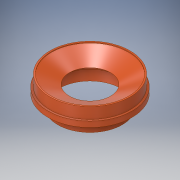
# Autodesk Inventor part: phenolic_top
Saved by Autodesk Inventor 2017 SP1 (Build 210196100, 196)
## iProperties
Created: 2016-07-25
Part Number: phenolic_top
Material: Phenolic Resin
Document SubType Name: Modeling
Designer: Jared
Density: 1.38 g/cm^3
Appearance: Smooth - Light Orange
Author: Jared
Autodesk Inventor part; units mm, degrees
ref_plane "YZ Plane" through (0, 0, 0) normal (1, 0, 0) x (0, 1, 0)
ref_plane "XZ Plane" through (0, 0, 0) normal (0, 1, 0) x (-1, 0, 0)
ref_plane "XY Plane" through (0, 0, 0) normal (0, 0, 1) x (1, 0, 0)
sketch "Sketch1" plane through (0, 0, 0) normal (0, 0, 1) x (1, 0, 0)
  line L0 (0, 25.4) -> (-28.702, 25.4) construction
  line L1 (0, 25.4) -> (-95.25, 25.4) construction
  line L2 (-95.25, 25.4) -> (-90.805, 25.4) construction
  line L3 (-90.805, 25.4) -> (-90.805, 22.4389) construction
  line L4 (-90.805, 0) -> (-95.25, 0)
  line L5 (-28.702, 59.6457) -> (-28.702, -91.9304) construction
  arc A0 (-28.9184, -9.248) -> (-32.3684, -1.8494) centre (-35.052, -7.6045) ccw
  line L6 (-76.2, -185.7054) -> (-28.702, -8.4405)
  line L7 (-90.805, 25.4) -> (-90.805, 0)
  line L8 (-87.63, 23.9195) -> (-32.3684, -1.8494)
  line L9 (-28.702, -7.6045) -> (-60.452, -7.6045) construction
  line L10 (-60.452, -126.9331) -> (-54.102, -126.9331) construction
  line L11 (-54.102, -126.9331) -> (-54.102, -103.2346) construction
  line L12 (-54.102, -103.2346) -> (-60.452, -103.2346)
  line L13 (-60.452, 11.2462) -> (-60.452, 1.7212) construction
  line L14 (-60.452, 11.2462) -> (-60.452, 4.7154) construction
  line L15 (-60.452, 4.7154) -> (-46.4468, 4.7154)
  line L16 (-95.25, 0) -> (-95.25, -12.7) construction
  line L17 (-60.452, -12.7) -> (-73.152, -12.7) construction
  line L18 (-95.25, -12.7) -> (-95.25, -25.4) construction
  line L19 (-95.25, -25.4) -> (-95.25, -88.9) construction
  line L20 (-95.25, -88.9) -> (-82.55, -88.9) construction
  line L21 (-82.55, -88.9) -> (-82.55, -25.4) construction
  line L22 (-95.25, -25.4) -> (-82.55, -25.4)
  line L23 (-82.55, -25.4) -> (-82.55, -88.9)
  line L24 (-82.55, -88.9) -> (-95.25, -88.9)
  line L25 (-95.25, -12.7) -> (-73.152, -12.7)
  line L26 (-73.152, -138.7824) -> (-63.627, -138.7824)
  line L27 (-82.55, -88.9) -> (-82.55, -185.7054)
  line L28 (-82.55, -185.7054) -> (-76.2, -185.7054)
  line L29 (-73.152, -12.7) -> (-73.152, -138.7824)
  line L30 (-88.9, -25.4) -> (-88.9, -31.3436)
  line L31 (-88.9, -31.3436) -> (-95.25, -31.3436)
  line L32 (-95.25, 0) -> (-95.25, -25.4)
  line L33 (-95.25, -31.3436) -> (-95.25, -88.9)
  line L34 (-88.9, -160.3054) -> (-88.9, -221.2532)
  line L35 (-28.9184, -9.248) -> (-85.725, -221.2532)
  line L36 (-85.725, -221.2532) -> (-88.9, -221.2532)
  line L37 (-82.55, -160.3054) -> (-88.9, -160.3054)
  line L38 (-66.802, -38.1) -> (-66.802, 4.7154)
  line L39 (-66.802, 4.7154) -> (-60.452, 4.7154)
  line L40 (-66.802, -38.1) -> (-60.452, -103.2346)
  line L41 (-60.452, 11.2462) -> (-60.452, 4.7154) construction
  line L42 (-60.452, -7.6045) -> (-60.452, -12.7) construction
  line L43 (-60.452, -103.2346) -> (-60.452, -126.9331) construction
  line L44 (0, 59.6457) -> (0, -91.9304) construction
  line L45 (-73.152, -38.1) -> (-69.977, -38.1)
  line L46 (-69.977, -38.1) -> (-69.977, -12.7)
  line L47 (-66.802, -12.7) -> (-69.977, -12.7)
  line L48 (-90.805, 25.4) -> (-87.63, 25.4)
  line L49 (-87.63, 25.4) -> (-87.63, 23.9195)
  point P0 (0, 0)
  point P1 (-95.25, -255.9127)
  point P2 (-88.7095, 22.4389)
  dimension "d0" = 28.702
  dimension "d1" = 95.25
  dimension "d2" = 4.445
  dimension "d5" = 25.4
  dimension "d6" = 25.4
  dimension "d8" = 12.7
  dimension "d12" = 31.75
  dimension "d13" = 6.35
  dimension "d16" = 12.7
  dimension "d17" = 12.7
  dimension "d18" = 12.7
  dimension "d19" = 63.5
  dimension "d20" = 12.7
  dimension "d22" = 9.525
  dimension "d23" = 6.35
  dimension "d25" = 5.9436
  dimension "d27" = 3.175
  dimension "d28" = 6.35
  dimension "d29" = 25.4
  dimension "d30" = 107.95
  dimension "d31" = 6.35
  dimension "d33" = 20.3552
  dimension "d34" = 15
  dimension "d35" = 3.175
  dimension "d36" = 25.4
  dimension "d38" = 3.175
  dimension "d39" = 1.4805
  dimension "d40" = 25
  constraints: 100 end point, 27 perpendicular, 20 point on line, 16 vertical, 5 vertical alignment, 4 horizontal, 4 tangent, 3 midpoint, 3 point on circle, 2 collinear, 1 centre point, 1 horizontal alignment
  measures "d0" distance of L0.start L0.end
  measures "d1" distance of L0.start L1.end
  measures "d2" distance of L2.end L1.end
  measures "d5" distance of point (0, 0) L0.start
  measures "d6" distance of L2.end L4.start
  measures "d8" diameter of A0
  measures "d12" distance of L9.end L9.start
  measures "d13" distance of L10.start L10.end
  measures "d16" distance of L4.end L16.end
  measures "d17" distance of L17.start L17.end
  measures "d18" distance of L16.end L18.end
  measures "d19" distance of L19.end L18.end
  measures "d20" distance of L19.end L20.end
  measures "d22" distance of L26.start L26.end
  measures "d23" distance of L27.end L6.start
  measures "d25" distance of L30.start L30.end
  measures "d27" distance of L34.end L35.end
  measures "d28" distance of L37.start L34.start
  measures "d29" distance from line of L27.end L37
  measures "d30" distance of L12.end L14.end
  measures "d31" distance between parallel lines of L29 L38
  measures "d33" distance of L15.end L38.end
  measures "d34" angle of L5 L35
  measures "d35" distance of L47.start L46.end
  measures "d36" distance from line of L17.end L45
  measures "d38" distance between parallel lines of L3 L49
  measures "d39" distance of L48.end L8.start
  measures "d40" angle of L1 L8
revolve "Revolution1" add sketch "Sketch1" angle 360 about axis through (0, 59.6457, 0) along (0, -1, 0) contours L7 L48 L49 L8 L15 L39 L38 L47 L46 L45 L29 L25 L32 L4
body "Solid1"
